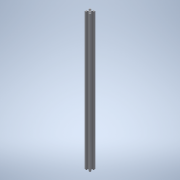
# Autodesk Inventor part: 20mm_V-Rail_Extrusion Template
Saved by Autodesk Inventor 2022.1 (Build 261234020, 234B)
## iProperties
Material: 6105-T5 Aluminum
Company: 80/20 Inc.
Created: 2014-04-23
Part Number: 20mm_V-Rail_Extrusion Template
Material: Aluminum 6105 T-5
Document SubType Name: Modeling
Designer: Ross Bowman
Density: 2.71 g/cm^3
Engineer: Ross Bowman
Catalog Web Link: 8020.net
Vendor: 80/20 Inc.
Mass: 43.1913 g
Surface Area: 184.633 cm^2
Volume: 15.9377 cm^3
Appearance: Aluminum - Flat
Author: Ross Bowman
Keywords: 80/20 , 8020 , T-Slot , Extrusion
Autodesk Inventor part; units mm, degrees
ref_plane "YZ Plane" through (0, 0, 0) normal (1, 0, 0) x (0, 1, 0)
ref_plane "XZ Plane" through (0, 0, 0) normal (0, 1, 0) x (-1, 0, 0)
ref_plane "XY Plane" through (0, 0, 0) normal (0, 0, 1) x (1, 0, 0)
sketch "Sketch1" plane through (0, 0, 0) normal (0, 0, 1) x (1, 0, 0)
  circle A0 centre (0, 0) radius 2.5
  line L0 (-9.9932, 4.515) -> (-7.9864, 3.0135)
  line L1 (-7.486, 6.0081) -> (-7.2469, 6.008)
  line L2 (-6.8934, 5.8613) -> (-4.8771, 3.8419)
  arc A1 (-6.8934, 5.8613) -> (-7.2469, 6.008) centre (-7.2472, 5.508) ccw
  circle A2 centre (0, 0) radius 2.5
  line L3 (-9.9932, 4.515) -> (-9.9932, 9.9932)
  line L4 (-7.9864, 3.0135) -> (-7.9864, 5.5081)
  arc A3 (-7.486, 6.0081) -> (-7.9864, 5.5081) centre (-7.4864, 5.5081) ccw
  line L5 (-4, 1.7222) -> (-4, 0)
  line L6 (-9.9932, -4.515) -> (-7.9864, -3.0135)
  line L7 (-6.8934, -5.8613) -> (-4.8771, -3.8419)
  arc A4 (-7.2469, -6.008) -> (-6.8934, -5.8613) centre (-7.2472, -5.508) ccw
  line L8 (-7.486, -6.0081) -> (-7.2469, -6.008)
  line L9 (-9.9932, -4.515) -> (-9.9932, -9.9932)
  line L10 (-7.9864, -3.0135) -> (-7.9864, -5.5081)
  arc A5 (-7.9864, -5.5081) -> (-7.486, -6.0081) centre (-7.4864, -5.5081) ccw
  line L11 (-4, -1.7222) -> (-4, 0)
  line L12 (9.9932, 4.515) -> (7.9864, 3.0135)
  line L13 (6.8934, 5.8613) -> (4.8771, 3.8419)
  arc A6 (7.2469, 6.008) -> (6.8934, 5.8613) centre (7.2472, 5.508) ccw
  line L14 (7.486, 6.0081) -> (7.2469, 6.008)
  line L15 (9.9932, 4.515) -> (9.9932, 9.9932)
  line L16 (7.9864, 3.0135) -> (7.9864, 5.5081)
  arc A7 (7.9864, 5.5081) -> (7.486, 6.0081) centre (7.4864, 5.5081) ccw
  line L17 (4, 1.7222) -> (4, 0)
  line L18 (9.9932, -4.515) -> (7.9864, -3.0135)
  line L19 (6.8934, -5.8613) -> (4.8771, -3.8419)
  arc A8 (6.8934, -5.8613) -> (7.2469, -6.008) centre (7.2472, -5.508) ccw
  line L20 (7.486, -6.0081) -> (7.2469, -6.008)
  line L21 (9.9932, -4.515) -> (9.9932, -9.9932)
  line L22 (7.9864, -3.0135) -> (7.9864, -5.5081)
  arc A9 (7.486, -6.0081) -> (7.9864, -5.5081) centre (7.4864, -5.5081) ccw
  line L23 (4, -1.7222) -> (4, 0)
  circle A10 centre (0, 0) radius 2.5
  line L24 (-4.515, -9.9932) -> (-3.0135, -7.9864)
  line L25 (-5.8613, -6.8934) -> (-3.8419, -4.8771)
  arc A11 (-5.8613, -6.8934) -> (-6.008, -7.2469) centre (-5.508, -7.2472) ccw
  line L26 (-6.0081, -7.486) -> (-6.008, -7.2469)
  circle A12 centre (0, 0) radius 2.5
  line L27 (-4.515, -9.9932) -> (-9.9932, -9.9932)
  line L28 (-3.0135, -7.9864) -> (-5.5081, -7.9864)
  arc A13 (-6.0081, -7.486) -> (-5.5081, -7.9864) centre (-5.5081, -7.4864) ccw
  line L29 (-1.7222, -4) -> (0, -4)
  line L30 (4.515, -9.9932) -> (3.0135, -7.9864)
  line L31 (5.8613, -6.8934) -> (3.8419, -4.8771)
  arc A14 (6.008, -7.2469) -> (5.8613, -6.8934) centre (5.508, -7.2472) ccw
  line L32 (6.0081, -7.486) -> (6.008, -7.2469)
  line L33 (4.515, -9.9932) -> (9.9932, -9.9932)
  line L34 (3.0135, -7.9864) -> (5.5081, -7.9864)
  arc A15 (5.5081, -7.9864) -> (6.0081, -7.486) centre (5.5081, -7.4864) ccw
  line L35 (1.7222, -4) -> (0, -4)
  line L36 (-1.7222, 4) -> (0, 4)
  line L37 (1.7222, 4) -> (0, 4)
  line L38 (5.8613, 6.8934) -> (3.8419, 4.8771)
  arc A16 (5.8613, 6.8934) -> (6.008, 7.2469) centre (5.508, 7.2472) ccw
  line L39 (6.0081, 7.486) -> (6.008, 7.2469)
  line L40 (3.0135, 7.9864) -> (5.5081, 7.9864)
  arc A17 (6.0081, 7.486) -> (5.5081, 7.9864) centre (5.5081, 7.4864) ccw
  line L41 (4.515, 9.9932) -> (3.0135, 7.9864)
  line L42 (4.515, 9.9932) -> (9.9932, 9.9932)
  line L43 (-5.8613, 6.8934) -> (-3.8419, 4.8771)
  arc A18 (-6.008, 7.2469) -> (-5.8613, 6.8934) centre (-5.508, 7.2472) ccw
  line L44 (-6.0081, 7.486) -> (-6.008, 7.2469)
  line L45 (-3.0135, 7.9864) -> (-5.5081, 7.9864)
  arc A19 (-5.5081, 7.9864) -> (-6.0081, 7.486) centre (-5.5081, 7.4864) ccw
  line L46 (-4.515, 9.9932) -> (-3.0135, 7.9864)
  line L47 (-4.515, 9.9932) -> (-9.9932, 9.9932)
  arc A20 (1.7222, 4) -> (3.8419, 4.8771) centre (1.7222, 7) ccw
  arc A21 (-3.8419, 4.8771) -> (-1.7222, 4) centre (-1.7222, 7) ccw
  arc A22 (-4, 1.7222) -> (-4.8771, 3.8419) centre (-7, 1.7222) ccw
  arc A23 (-4.8771, -3.8419) -> (-4, -1.7222) centre (-7, -1.7222) ccw
  arc A24 (-1.7222, -4) -> (-3.8419, -4.8771) centre (-1.7222, -7) ccw
  arc A25 (3.8419, -4.8771) -> (1.7222, -4) centre (1.7222, -7) ccw
  arc A26 (4, -1.7222) -> (4.8771, -3.8419) centre (7, -1.7222) ccw
  arc A27 (4.8771, 3.8419) -> (4, 1.7222) centre (7, 1.7222) ccw
  point P0 (-7.9864, 6.0085)
  point P1 (-7.9864, -6.0085)
  point P2 (7.9864, 6.0085)
  point P3 (7.9864, -6.0085)
  point P4 (-6.0085, -7.9864)
  point P5 (6.0085, -7.9864)
  point P6 (6.0085, 7.9864)
  point P7 (-6.0085, 7.9864)
  constraints: 96 end point, 48 point on circle, 28 centre point, 16 point on line
extrude "Extrusion9" add sketch "Sketch1" along normal blind 527.05
body "Solid3"
